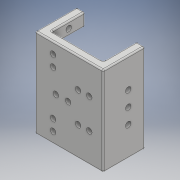
# Autodesk Inventor part: holder
Saved by Autodesk Inventor 2018 (Build 220112000, 112)
## iProperties
Created: 2018-04-27
Part Number: holder
Material: Generic
Document SubType Name: Modeling
Designer: Matyi
Density: 1 g/cm^3
Appearance: Default
Author: Matyi
Autodesk Inventor part; units mm, degrees
ref_plane "YZ Plane" through (0, 0, 0) normal (1, 0, 0) x (0, 1, 0)
ref_plane "XZ Plane" through (0, 0, 0) normal (0, 1, 0) x (-1, 0, 0)
ref_plane "XY Plane" through (0, 0, 0) normal (0, 0, 1) x (1, 0, 0)
sketch "Sketch1" plane through (0, 0, 0) normal (0, 1, 0) x (-1, 0, 0)
  line L0 (0, 0) -> (24.5, 0)
  line L1 (24.5, 0) -> (24.5, -32)
  line L2 (24.5, -32) -> (0, -32)
  line L3 (0, -32) -> (0, 0)
  line L4 (24.5, 0) -> (21.5, 0)
  line L5 (21.5, 0) -> (21.5, -4.7)
  line L6 (21.5, -4.7) -> (24.5, -4.7)
  line L7 (24.5, -4.7) -> (24.5, 0)
  line L8 (24.5, -32) -> (21.5, -32)
  line L9 (21.5, -32) -> (21.5, -27.3)
  line L10 (21.5, -27.3) -> (24.5, -27.3)
  line L11 (24.5, -27.3) -> (24.5, -32)
  line L12 (0, 0) -> (3, 0)
  line L13 (3, 0) -> (3, -32)
  line L14 (3, -32) -> (0, -32)
  line L15 (0, -32) -> (0, 0)
  circle A0 centre (18, -4) radius 1
  circle A1 centre (18, -8) radius 1
  circle A2 centre (18, -24) radius 1
  circle A3 centre (18, -28) radius 1
  circle A4 centre (9, -10.6) radius 1
  circle A5 centre (5, -10.6) radius 1
  circle A6 centre (9, -21.4) radius 1
  circle A7 centre (5, -21.4) radius 1
  circle A8 centre (17, -16) radius 1
  circle A9 centre (12.6, -16) radius 1
  dimension "d0" = 24.5
  dimension "d1" = 32
  dimension "d2" = 3
  dimension "d3" = 4.7
  dimension "d4" = 4.7
  dimension "d5" = 3
  dimension "d6" = 2
  dimension "d7" = 2
  dimension "d8" = 2
  dimension "d9" = 2
  dimension "d10" = 2
  dimension "d11" = 2
  dimension "d12" = 2
  dimension "d13" = 2
  dimension "d14" = 2
  dimension "d15" = 2
  dimension "d16" = 4
  dimension "d17" = 4
  dimension "d18" = 4
  dimension "d19" = 4
  dimension "d20" = 18
  dimension "d21" = 18
  dimension "d22" = 18
  dimension "d23" = 18
  dimension "d24" = 5
  dimension "d25" = 4
  dimension "d26" = 5
  dimension "d27" = 4
  dimension "d28" = 10.6
  dimension "d29" = 10.6
  dimension "d30" = 10.6
  dimension "d31" = 10.6
  dimension "d32" = 16
  dimension "d33" = 16
  dimension "d34" = 4.4
  dimension "d35" = 12.6
  dimension "d36" = 3
  constraints: 32 end point, 10 centre point, 8 parallel, 4 horizontal, 4 perpendicular, 1 point on line
  measures "d0" distance of L1.end L2.end
  measures "d1" distance of L0.end L1.end
  measures "d2" distance of L6.end L5.end
  measures "d3" distance of L5.end L4.end
  measures "d4" distance of L8.end L9.end
  measures "d5" distance of L13.end L14.end
  measures "d6" diameter of A0
  measures "d7" diameter of A1
  measures "d8" diameter of A2
  measures "d9" diameter of A3
  measures "d10" diameter of A4
  measures "d11" diameter of A5
  measures "d12" diameter of A6
  measures "d13" diameter of A7
  measures "d14" diameter of A8
  measures "d15" diameter of A9
  measures "d16" distance from line of L0 A0.centre
  measures "d17" distance of A1.centre A0.centre
  measures "d18" distance from line of L2 A3.centre
  measures "d19" distance of A3.centre A2.centre
  measures "d20" distance from line of L3 A3.centre
  measures "d21" distance from line of L3 A2.centre
  measures "d22" distance from line of L3 A1.centre
  measures "d23" distance from line of L15 A0.centre
  measures "d24" distance from line of L15 A5.centre
  measures "d25" distance of A5.centre A4.centre
  measures "d26" distance from line of L3 A7.centre
  measures "d27" distance of A7.centre A6.centre
  measures "d28" distance from line of L0 A4.centre
  measures "d29" distance from line of L0 A5.centre
  measures "d30" distance from line of L2 A6.centre
  measures "d31" distance from line of L2 A7.centre
  measures "d32" distance from line of L2 A8.centre
  measures "d33" distance from line of L2 A9.centre
  measures "d34" distance of A9.centre A8.centre
  measures "d35" distance from line of L15 A9.centre
  measures "d36" distance between parallel lines of L1 L9
extrude "Extrusion1" add sketch "Sketch1" along normal blind 3 contours L0 L5 L6 L1 L10 L9 L2 L13
extrude "Extrusion2" add sketch "Sketch1" along normal blind 15 contours L0 L13 L2 L3 | L0 L1 L6 L5 | L9 L10 L1 L2
sketch "Sketch2" plane through (-24.5, 0, -32) normal (-1, 0, 0) x (0, 0, 1)
  circle A0 centre (29.7, 9.1) radius 1
  circle A1 centre (2.3, 9.1) radius 1
  line L0 (27.3, 15) -> (32, 15) projected
  line L1 (0, 15) -> (4.7, 15) projected
  line L2 (32, 0) -> (32, 15) projected
  line L3 (0, 0) -> (0, 15) projected
  dimension "d41" = 2
  dimension "d42" = 2
  dimension "d43" = 5.9
  dimension "d44" = 5.9
  dimension "d45" = 2.3
  dimension "d46" = 2.3
  constraints: 2 centre point
  measures "d41" diameter of A0
  measures "d42" diameter of A1
  measures "d43" distance from line of L0 A0.centre
  measures "d44" distance from line of L1 A1.centre
  measures "d45" distance from line of L2 A0.centre
  measures "d46" distance from line of L3 A1.centre
extrude "Extrusion3" cut sketch "Sketch2" against normal blind 3
sketch "Sketch3" plane through (0, 0, 0) normal (1, 0, 0) x (0, 0, -1)
  circle A0 centre (10.6, 9) radius 1
  circle A1 centre (21.4, 9) radius 1
  line L0 (0, 15) -> (32, 15) projected
  line L1 (32, 0) -> (32, 15) projected
  line L2 (0, 0) -> (0, 15) projected
  circle A2 centre (16, 9) radius 1
  dimension "d51" = 2
  dimension "d52" = 2
  dimension "d53" = 6
  dimension "d54" = 10.6
  dimension "d55" = 6
  dimension "d56" = 10.6
  dimension "d60" = 2
  dimension "d61" = 6
  dimension "d62" = 16
  constraints: 3 centre point
  measures "d51" diameter of A0
  measures "d52" diameter of A1
  measures "d53" distance from line of L0 A1.centre
  measures "d54" distance from line of L1 A1.centre
  measures "d55" distance from line of L0 A0.centre
  measures "d56" distance from line of L2 A0.centre
  measures "d60" diameter of A2
  measures "d61" distance from line of L0 A2.centre
  measures "d62" distance from line of L1 A2.centre
extrude "Extrusion4" cut sketch "Sketch3" against normal blind 3 contours A0 | A1
fillet "Fillet3" radius 0.5 36 edges at (-24.5, 9, -4.7) (-24.5, 7.5, 0) (-24.5, 15, -2.35) (-24.5, 3, -16) (-24.5, 0, -16) (-24.5, 9, -27.3) (-24.5, 15, -29.65) (-24.5, 7.5, -32) (-12.25, 0, -32) (-12.25, 3, 0) (-23, 3, -4.7) (-23, 15, -4.7) (-23, 15, 0) (-23, 15, -27.3) (-23, 15, -32) (-23, 3, -27.3) (-12.25, 0, 0) (-21.5, 9, 0) (-21.5, 15, -2.35) (-21.5, 9, -27.3) (-21.5, 15, -29.65) (-21.5, 9, -32) (-21.5, 9, -4.7) (-21.5, 3, -2.35) (-21.5, 3, -29.65) (-12.25, 3, -32) (-3, 3, -16) (0, 0, -16) (-3, 9, -32) (0, 7.5, -32) (-1.5, 15, -32) (-3, 15, -16) (0, 15, -16) (-1.5, 15, 0) (-3, 9, 0) (0, 7.5, 0)
extrude "Extrusion5" cut sketch "Sketch3" against normal blind 3 contours A2
body "Solid1"
